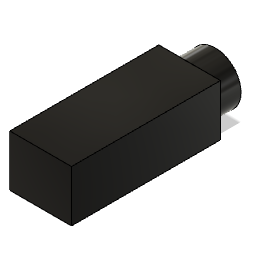
SJ-3523-SMT-TR (Autodesk Fusion 360 design; units mm, degrees)
Autodesk Fusion 360 part; units mm, degrees
sketch "Sketch1" plane through (0, 0, 0) normal (0, 1, 0) x (1, 0, 0)
  line L0 (3, -7.25) -> (-3, -7.25)
  line L1 (-3, -7.25) -> (-3, 7.25)
  line L2 (-3, 7.25) -> (3, 7.25)
  line L3 (3, 7.25) -> (3, -7.25)
  line L4 (3, -7.25) -> (-3, 7.25) construction
  line L5 (-3, -7.25) -> (3, 7.25) construction
  dimension "d1" = 14.5
  dimension "d2" = 6
  constraint perpendicular L0 L1
  constraint parallel L0 L2
  constraint parallel L1 L3
  constraint horizontal L0
  constraint coincident L4 origin
  constraint coincident L5 origin
  measures "d1" distance of L0.start L2.end
  measures "d2" distance of L1.end L2.end
extrude "Extrude1" add sketch "Sketch1" along normal blind 5
sketch "Sketch2" plane through (0, 0, -7.25) normal (0, 0, -1) x (-1, 0, 0)
  line L0 (-3, 0) -> (3, 0)
  line L1 (3, 0) -> (3, 5)
  line L2 (3, 5) -> (-3, 5)
  line L3 (-3, 5) -> (-3, 0)
  line L4 (-3, 5) -> (3, 0) construction
  circle A0 centre (0, 2.5) radius 2.5
  dimension "d5" = 5
  constraint coincident L2.end L3.start
  constraint coincident L0.end L1.start
  constraint midpoint L4 A0.centre
  measures "d5" diameter of A0
extrude "Extrude2" add sketch "Sketch2" along normal blind 2.5 contours A0
named bodies: "SJ-3523-SMT-TR"
